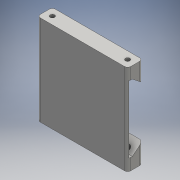
# Autodesk Inventor part: 60x60CameraMountSlim
Saved by Autodesk Inventor 2016 (Build 200138000, 138)
## iProperties
Created: 2016-05-22
Part Number: 60x60CameraMountSlim
Material: Generic
Document SubType Name: Modeling
Designer: Kurtis
Density: 1 g/cm^3
Appearance: Default
Author: Kurtis
Autodesk Inventor part; units mm, degrees
ref_plane "YZ Plane" through (0, 0, 0) normal (1, 0, 0) x (0, 1, 0)
ref_plane "XZ Plane" through (0, 0, 0) normal (0, 1, 0) x (-1, 0, 0)
ref_plane "XY Plane" through (0, 0, 0) normal (0, 0, 1) x (1, 0, 0)
sketch "Sketch1" plane through (0, 0, 0) normal (0, 0, 1) x (1, 0, 0)
  line L0 (30, -30) -> (30, 30)
  line L1 (30, 30) -> (-30, 30)
  line L2 (-30, 30) -> (-30, -30)
  line L3 (-30, -30) -> (30, 30) construction
  line L4 (30, -30) -> (-30, 30) construction
  line L5 (30, 30) -> (25, 30) construction
  line L6 (25, 30) -> (25, 25) construction
  line L7 (-30, 30) -> (-25, 30) construction
  line L8 (-25, 30) -> (-25, 25) construction
  line L9 (-30, -30) -> (-30, -25) construction
  line L10 (-30, -25) -> (-25, -25) construction
  line L11 (30, -30) -> (30, -25) construction
  line L12 (30, -25) -> (25, -25) construction
  circle A0 centre (-25, 25) radius 1.5
  circle A1 centre (25, 25) radius 1.5
  circle A2 centre (25, -25) radius 1.5
  circle A3 centre (-25, -25) radius 1.5
  line L13 (30, 30) -> (30, 20) construction
  line L14 (30, 20) -> (-30, 20)
  point P0 (0, 0)
  dimension "d0" = 60
  dimension "d1" = 60
  dimension "d2" = 5
  dimension "d3" = 5
  dimension "d4" = 5
  dimension "d5" = 5
  dimension "d6" = 5
  dimension "d7" = 5
  dimension "d8" = 5
  dimension "d9" = 5
  dimension "d10" = 3
  dimension "d11" = 3
  dimension "d12" = 3
  dimension "d13" = 3
  dimension "d46" = 10
  constraints: 30 end point, 10 point on line, 4 centre point, 4 coincident, 2 midpoint, 1 parallel, 1 perpendicular
  measures "d0" distance of L1.end L0.end
  measures "d1" distance of L0.end L0.start
  measures "d2" distance of L0.end L5.end
  measures "d3" distance of L5.end L6.end
  measures "d4" distance of L1.end L7.end
  measures "d5" distance of L7.end L8.end
  measures "d6" distance of L2.end L9.end
  measures "d7" distance of L9.end L10.end
  measures "d8" distance of L0.start L11.end
  measures "d9" distance of L11.end L12.end
  measures "d10" diameter of A0
  measures "d11" diameter of A1
  measures "d12" diameter of A2
  measures "d13" diameter of A3
  measures "d46" distance of L0.end L13.end
extrude "Block" add sketch "Sketch1" along normal blind 60 contours L14 L2 L1 L0
sketch "Sketch2" plane through (30, -30, 0) normal (1, 0, 0) x (0, 0, -1)
  line L0 (0, 60) -> (-60, 60) projected
  line L1 (-30, 60) -> (-13.25, 60)
  line L2 (-30, 60) -> (-46.75, 60)
  line L3 (-30, 60) -> (-30, 51.1) construction
  line L4 (-30, 51.1) -> (-7.75, 51.1)
  line L5 (-30, 51.1) -> (-52.25, 51.1)
  line L6 (-52.25, 51.1) -> (-52.25, 53.1)
  line L7 (-7.75, 51.1) -> (-7.75, 53.1)
  line L8 (-7.75, 53.1) -> (-13.25, 60)
  line L9 (-52.25, 53.1) -> (-46.75, 60)
  point P0 (0, 30)
  dimension "d17" = 16.75
  dimension "d18" = 16.75
  dimension "d19" = 8.9
  dimension "d20" = 22.25
  dimension "d21" = 22.25
  dimension "d22" = 2
  dimension "d23" = 2
  constraints: 18 end point, 2 perpendicular, 2 point on line, 2 vertical, 1 horizontal, 1 midpoint
  measures "d17" distance of L1.start L1.end
  measures "d18" distance of L1.start L2.end
  measures "d19" distance of L1.start L3.end
  measures "d20" distance of L3.end L4.end
  measures "d21" distance of L3.end L5.end
  measures "d22" distance of L5.end L6.end
  measures "d23" distance of L4.end L7.end
extrude "Tripod Slot" cut sketch "Sketch2" against normal blind 60
sketch "Sketch3" plane through (0, 0, 60) normal (0, 0, 1) x (1, 0, 0)
  circle A0 centre (-25, -25) radius 1.5 construction
  line L0 (-25, -25) -> (-25, -20) construction
  line L1 (-25, -25) -> (-20, -25) construction
  line L2 (25.1388, -25) -> (25.1388, -20) construction
  line L3 (25.1388, -25) -> (30.1388, -25) construction
  line L4 (-25, 24.9661) -> (-25, 17.4661) construction
  line L5 (-25, 24.9661) -> (-17.5, 24.9661) construction
  line L6 (25.1388, 24.9661) -> (25.1388, 17.4661) construction
  line L7 (25.1388, 24.9661) -> (32.6388, 24.9661) construction
  line L8 (25.1388, 17.4661) -> (30, 17.4661) construction
  line L9 (30, 30) -> (30, 20) construction
  line L10 (-25, 17.4661) -> (-30, 17.4661) construction
  line L11 (-30, 30) -> (-30, 20) construction
  line L12 (-25, -20) -> (-30, -20) construction
  line L13 (25.1388, -20) -> (30, -20) construction
  line L14 (30, 17.4661) -> (5, 17.4661)
  line L15 (30, -20) -> (5, -20)
  line L16 (5, -20) -> (5, 17.4661)
  line L17 (-30, 17.4661) -> (-5, 17.4661)
  line L18 (-30, -20) -> (-5, -20)
  line L19 (-5, -20) -> (-5, 17.4661)
  line L20 (-30, 17.4661) -> (-30, -20)
  line L21 (30, 17.4661) -> (30, -20)
  point P0 (0, 0)
  point P1 (30, -30)
  point P2 (-30, -30)
  dimension "d26" = 5
  dimension "d27" = 90
  dimension "d28" = 5
  dimension "d29" = 90
  dimension "d30" = 7.5
  dimension "d31" = 90
  dimension "d32" = 7.5
  dimension "d33" = 90
  dimension "d34" = 25
  dimension "d35" = 25
  dimension "d36" = 25
  dimension "d37" = 25
  dimension "d38" = 90
  dimension "d39" = 90
  dimension "d40" = 4.8612
  dimension "d41" = 4.8612
  dimension "d42" = 55
  constraints: 40 end point, 7 perpendicular, 7 point on line, 6 horizontal, 4 vertical, 1 collinear, 1 parallel
  measures "d26" distance of L0.start L0.end
  measures "d27" angle of L1 L0
  measures "d28" distance of L2.start L2.end
  measures "d29" angle of L3 L2
  measures "d30" distance of L4.start L4.end
  measures "d31" angle of L4 L5
  measures "d32" distance of L6.start L6.end
  measures "d33" angle of L6 L7
  measures "d34" distance of L8.end L14.end
  measures "d35" distance of L13.end L15.end
  measures "d36" distance of L10.end L17.end
  measures "d37" distance of L12.end L18.end
  measures "d38" angle of L13 L9
  measures "d39" angle of L14 L19
  measures "d40" distance between parallel lines of L9 L2
  measures "d41" distance between parallel lines of L6 L9
  measures "d42" distance between parallel lines of L4 L9
extrude "Plastic Thinning" cut sketch "Sketch3" against normal blind 60
fillet "Strength" [suppressed]
fillet "Fillet3" radius 2 6 edges at (30, 20, 30) (30, 30, 6.625) (30, 30, 53.375) (-30, 20, 30) (-30, 30, 6.625) (-30, 30, 53.375)
body "Solid1"
